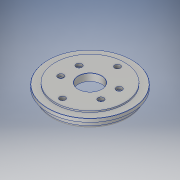
# Autodesk Inventor part: 2016.06.09 ps Hamamatsu PMT Adapter
Saved by Autodesk Inventor 2017 (Build 210142000, 142)
## iProperties
Created: 2016-06-09
Part Number: 2016.06.09 ps Hamamatsu PMT Adapter
Material: Aluminum 6061
Document SubType Name: Modeling
Designer: Darien Morrow
Density: 2.7 g/cm^3
Appearance: Aluminum - Flat
Author: Darien Morrow
Autodesk Inventor part; units mm, degrees
ref_plane "YZ Plane" through (0, 0, 0) normal (1, 0, 0) x (0, 1, 0)
ref_plane "XZ Plane" through (0, 0, 0) normal (0, 1, 0) x (-1, 0, 0)
ref_plane "XY Plane" through (0, 0, 0) normal (0, 0, 1) x (1, 0, 0)
sketch "Sketch1" plane through (0, 0, 0) normal (0, 0, 1) x (1, 0, 0)
  line L0 (17.5514, 0) -> (46.0756, 0)
  line L1 (46.0756, 0) -> (46.0756, 12.7)
  line L2 (46.0756, 12.7) -> (0, 12.7)
  line L3 (0, 12.7) -> (0, 0)
  line L4 (17.5514, 12.7) -> (17.5514, 0)
  line L5 (46.0756, 8.9662) -> (42.3672, 8.9662)
  line L6 (42.3672, 7.747) -> (42.3672, 0)
  line L7 (46.0756, 7.747) -> (42.3672, 7.747)
  line L8 (46.0756, 8.9662) -> (42.3672, 7.747)
  line L9 (0, 11.1252) -> (0, 12.7)
  line L10 (17.5514, 0) -> (23.85, 0)
  line L11 (0, -2.5) -> (0, 0)
  line L12 (0, 12.7) -> (38.0365, 12.7)
  line L13 (38.0365, 12.7) -> (38.0365, 14.2748)
  line L14 (38.0365, 14.2748) -> (0, 14.2748)
  line L15 (0, 14.2748) -> (0, 12.7)
  line L16 (17.5514, 12.7) -> (17.5514, 14.2748)
  line L17 (0, 0) -> (17.5514, 0)
  dimension "d1" = 12.7
  dimension "d3" = 3.7338
  dimension "d5" = 4.953
  dimension "d8" = 17.5514
  dimension "d9" = 42.3672
  dimension "d10" = 46.0756
  dimension "d11" = 1.5748
  dimension "d12" = 38.0365
  constraints: 36 end point, 7 perpendicular, 7 point on line, 4 horizontal, 4 parallel
  measures "d1" distance of L2.end L3.end
  measures "d3" distance between parallel lines of L5 L2
  measures "d5" distance between parallel lines of L7 L2
  measures "d8" distance between parallel lines of L4 L3
  measures "d9" distance between parallel lines of L6 L3
  measures "d10" distance between parallel lines of L1 L3
  measures "d11" distance between parallel lines of L2 L14
  measures "d12" distance between parallel lines of L13 L15
revolve "Revolution1" add sketch "Sketch1" angle 360 about axis through (0, 12.7, 0) along (0, -1, 0) contours L4 L2 L1 L8 L6 L0 | L17 L3 L2 L4 | L16 L14 L13 L2 | L2 L15 L14 L16
sketch "Sketch2" plane through (0, 14.2748, 0) normal (0, 1, 0) x (1, 0, 0)
  circle A0 centre (0, 0) radius 30.1752
  point P0 (0, 30.1752)
  point P1 (0, -30.1752)
  dimension "d14" = 60.3504
  constraints: 2 point on circle, 1 centre point, 1 coincident
  measures "d14" diameter of A0
hole "Hole1" at (0, 14.2748, -30.1752) at (0, 14.2748, 30.1752) direction (0, -1, 0) diameter 6.35 depth 7.62
fillet "Fillet1" radius 3.175 1 edges at (-42.3672, 0, 0)
sketch "Sketch3" plane through (0, 0, 0) normal (0, -1, 0) x (1, 0, 0)
  line L0 (27.305, 18.669) -> (-27.305, 18.669)
  line L1 (-28.575, 17.399) -> (-28.575, -17.399)
  line L2 (-27.305, -18.669) -> (27.305, -18.669)
  line L3 (28.575, -17.399) -> (28.575, 17.399)
  line L4 (28.575, 18.669) -> (-28.575, -18.669) construction
  line L5 (-28.575, 18.669) -> (28.575, -18.669) construction
  arc A0 (27.305, -18.669) -> (28.575, -17.399) centre (27.305, -17.399) ccw
  arc A1 (28.575, 17.399) -> (27.305, 18.669) centre (27.305, 17.399) ccw
  arc A2 (-27.305, 18.669) -> (-28.575, 17.399) centre (-27.305, 17.399) ccw
  arc A3 (-28.575, -17.399) -> (-27.305, -18.669) centre (-27.305, -17.399) ccw
  point P0 (0, 0)
  dimension "d23" = 57.15
  dimension "d24" = 37.338
  dimension "d25" = 1.27
  constraints: 12 end point, 8 point on circle, 8 point on line, 8 tangent, 4 centre point, 3 equal radius, 2 midpoint, 2 parallel, 1 horizontal, 1 perpendicular
  measures "d23" distance between parallel lines of L1 L3
  measures "d24" distance between parallel lines of L2 L0
  measures "d25" radius of A0
sketch "Sketch4" plane through (0, 14.2748, 0) normal (0, 1, 0) x (1, 0, 0)
  line L0 (21.9964, 9.9949) -> (-21.9964, 9.9949)
  line L1 (-21.9964, 9.9949) -> (-21.9964, -9.9949)
  line L2 (-21.9964, -9.9949) -> (21.9964, -9.9949)
  line L3 (21.9964, -9.9949) -> (21.9964, 9.9949)
  line L4 (21.9964, 9.9949) -> (-21.9964, -9.9949) construction
  line L5 (-21.9964, 9.9949) -> (21.9964, -9.9949) construction
  point P0 (0, 0)
  dimension "d26" = 19.9898
  dimension "d27" = 43.9928
  constraints: 12 end point, 4 coincident, 2 midpoint, 2 parallel, 1 horizontal, 1 perpendicular
  measures "d26" distance between parallel lines of L0 L2
  measures "d27" distance between parallel lines of L1 L3
hole "Hole2" at (21.9964, 14.2748, 9.9949) at (21.9964, 14.2748, -9.9949) at (-21.9964, 14.2748, 9.9949) at (-21.9964, 14.2748, -9.9949) direction (0, -1, 0) diameter 3.4036 end through all counterbore diameter 6.5024 counterbore depth 2.9972 clearance for "Socket Head Cap Screw" size "M3" standard "Ansi Metric M Profile"
extrude "Extrusion1" cut sketch "Sketch3" against normal blind 6.35
chamfer "Chamfer1" distance 0.508 angle 45 8 edges at (0, 0, 18.669) (28.203, 0, 18.297) (28.575, 0, 0) (28.203, 0, -18.297) (0, 0, -18.669) (-28.203, 0, -18.297) (-28.575, 0, 0) (-28.203, 0, 18.297)
sketch "Sketch5" plane through (0, 14.2748, 0) normal (0, 1, 0) x (1, 0, 0)
  circle A0 centre (0, 0) radius 12.7
  dimension "d40" = 25.4
  constraints: 1 centre point, 1 coincident
  measures "d40" diameter of A0
extrude "Extrusion2" cut sketch "Sketch5" against normal through all
chamfer "Chamfer2" distance 0.254 angle 45 2 edges at (-46.0756, 12.7, 0) (-12.7, 14.2748, 0)
body "Solid1"
